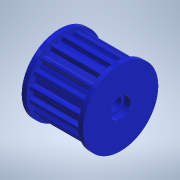
# Autodesk Inventor part: HTPT18S8M300-A-H12_b
Saved by Autodesk Inventor 2021 (Build 250183000, 183)
## iProperties
Category: PARTsolutions
Company: MISUMI
Part Number: HTPT18S8M300-A-H12_b
Material: ABS プラスチック
Catalog Web Link: www.cadenas.de
Description: HTPA__S8M150, HTPA__S8M250, HTPA__S8M300, HTPA__S8M400, HTPB__S8M150, HTPB__S8M250, HTPB__S8M300, HTPB__S8M400, HTPK__S8M150, HTPK__S8M250, HTPK__S8M300, HTPK__S8M400, HTPN__S8M150, HTPN__S8M250, HTPN__S8M300, HTPN__S8M400, HTPT__S8M150, HTPT__S8M250, HTPT__S8M300, HTPT__S8M400, HTPM__S8M150, HTPM__S8M250, HTPM__S8M300, HTPM__S8M400,_body-HTPP__S8M150, HTPP__S8M250, HTPP__S8M300, HTPP__S8M400 - High Torque Timing Pulleys S8M Type
Vendor: MISUMI
Document SubType Name: Modeling
Designer: partserver
Manufacturer: MISUMI
Mass: 50.873 g
Surface Area: 141.05 cm^2
Volume: 47.9934 cm^3
Density: 1.06 g/cm^3
Appearance: 青 - 壁塗料 - 光沢
PSOL_IDENT_0: {$CADENAS_DATA\23d-libs\misumi\metric\51_timing_pulleys\htpa_s8m.prj},749 {VTYP=3D},{NB=HTPT18S8M300
PSOL_IDENT_1: -A-H12_b},{LINA=HTPT18S8M300-A-H12},{NN=HTPA__S8M150, HTPA__S8M250, HTPA__S8M300, HTPA__S8M400, HTPB
PSOL_IDENT_2: __S8M150, HTPB__S8M250, HTPB__S8M300, HTPB__S8M400, HTPK__S8M150, HTPK__S8M250, HTPK__S8M300, HTPK__
PSOL_IDENT_3: S8M400, HTPN__S8M150, HTPN__S8M250, HTPN__S8M300, HTPN__S8M400, HTPT__S8M150, HTPT__S8M250, HTPT__S8
PSOL_IDENT_4: M300, HTPT__S8M400, HTPM__S8M150, HTPM__S8M250, HTPM__S8M300, HTPM__S8M400,_body},{DATE=17.01.2019 0
PSOL_IDENT_5: 4:07:40},{GEOMDATE=11.01.2019 07:18:36},{VERSION=},{LINEID=50},{WBVAR=MATP,ST,TNW,PS,SBS,DD,Z,J,Q,R,
PSOL_IDENT_6: S,T,ALT1,ALT2,M,QSC,QFC,QTC,ALT3,K,KSC,KFC,KTC,ALT4,ZM,ZSC,ZFC,ZTC,ALT5,ALT6,ALT7,FC,ALT8,SRG,ALT9,B
PSOL_IDENT_7: TC,TL,ALT10,TPC,ALT11,BC,ALT12,SLH},{WBNUMERIC=DD,Z,J,Q,R,S,T,QSC,QFC,QTC,K,KSC,KFC,KTC,ZSC,ZFC,ZTC,
PSOL_IDENT_8: FC,SRG,BTC,TL,BC,SLH}  {NB=HTPT18S8M300-A-H12_b},{LINA=HTPT18S8M300-A-H12},{KT=DUMMY},{PN=HTPT18S8M3
PSOL_IDENT_9: 00-A-H12},{TYPE=HTPT},{MATP=S45C},{MATPALG= 'A7075','A7075','S45C','1045 Carbon Steel Equivalent' },
PSOL_IDENT_10: {ST=-},{STALG= '-','-','BO','Black Oxide','ENP','Electroless Nickel Plating' },{NT=18},{TNW=S8M300},
PSOL_IDENT_11: {TNWALG= 'S8M150','S8M250','S8M300','S8M400' },{BW=30},{PS=A},{PSALG= 'A','B' },{SBS=H},{SBSALG= 'H'
PSOL_IDENT_12: ,'Round Hole','P','Round Hole + Tap','N','New JIS Keywayed Bore + Tap (Standard)','C','Old JIS Keywa
PSOL_IDENT_13: yed Bore + Tap','V','Stepped Hole','Y','Both Ends Stepped Hole','WB','Double Stepped Hole' },{DD=12.
PSOL_IDENT_14: 0},{DDALG=12.0,12.7,[13:32/1]},{DDHA=12.0,12.7,[13:32/1]},{DDPA=12.0,12.7,[13:26/1]},{DDNA=[12:26/1]
PSOL_IDENT_15: },{DDCA=[12,15,16,18,19,20]},{DDVA=12.0,12.7,[13:30/1]},{DDY=[12:30/1]},{DDWB=[12:28/1]},{DDHB=},{DD
PSOL_IDENT_16: PB=},{DDNB=},{DDCB=},{DDVFB=},{Z=0},{ZALG=[0]},{ZMIN=14.000},{ZAMAX=32.000},{ZBMAX=0.000},{DDZ=12.00
PSOL_IDENT_17: 0},{J=0.0},{JALG=[0]},{JMIN=3.000},{JMAX=35.000},{JPN=},{Q=0},{QALG=[0]},{QRMIN=14.000},{QRMAX=32.00
PSOL_IDENT_18: 0},{WBQMIN=16.000},{R=0},{RALG=[0]},{WBRMAX=-2.000},{S=0.0},{SALG=[0]},{SMAX=23.000},{T=0.0},{TALG=[
PSOL_IDENT_19: 0]},{TMAX=23.000},{SBSPN=-H12},{A=33},{W=38},{L=0},{PD=45.84},{OD=44.46},{D=0},{DALG=32.000},{DE=36.
PSOL_IDENT_20: 000},{F=52},{E=36},{TT=1.6},{BBK=0.000},{TTK=0.000},{ALT1=},{ALT1ALG= '','Not applicable' },{ANG=120
PSOL_IDENT_21: .000},{ALT1PN=},{ALT2=},{ALT2ALG= '','w/o Side Tapped Hole','QSC','with QSC (6 Places Side Tapped Ho
PSOL_IDENT_22: le)','QFC','with QFC (4 Places Side Tapped Hole)','QTC','with QTC (3 Places Side Tapped Hole)' },{M=
PSOL_IDENT_23: N/A},{MALG= 'N/A' },{MFTALG= 'N/A' },{MSALG= 'N/A' },{M3D=0.000},{KDML=0.000},{ML=0.000},{MUL=0.000}
PSOL_IDENT_24: ,{PITCH=0.000},{QSC=0.0},{QSCALG=0},{QFC=0.0},{QFCALG=0},{QTC=0.0},{QTCALG=0},{QPCDMIN=0.000},{QPCDM
PSOL_IDENT_25: INALG=0.000},{QPCDMAX=32.000},{ALT2PN=},{TAP=0.000},{ALT3=},{ALT3ALG= '','w/o Side Through Hole','KS
PSOL_IDENT_26: C','with KSC (6 Places Side Through Hole)','KFC','with KFC (4 Places Side Through Hole)','KTC','with
PSOL_IDENT_27: KTC (3 Places Side Through Hole)' },{K=0.0},{KALG=0},{KMIN=4.000},{KFTMAX=8.000},{KSMAX=8.000},{KSC=
PSOL_IDENT_28: 0.0},{KSCALG=0},{KFC=0.0},{KFCALG=0},{KTC=0.0},{KTCALG=0},{KSCMIN=16.000},{KPCDMIN=16.000},{KPCDMAX=
PSOL_IDENT_29: 32.000},{ALT3PN=},{ALT4=},{ALT4ALG= '','w/o Side Counterbored','ZSC','with ZSC (6 Places Side Counte
PSOL_IDENT_30: rbored)','ZFC','with ZFC (4 Places Side Counterbored)','ZTC','with ZTC (3 Places Side Counterbored)'
PSOL_IDENT_31: },{ALT4MIN=22.500},{ALT4MAX=25.500},{ZM=N/A},{ZMALG= 'N/A' },{ZMFTALG= 'N/A' },{ZMSALG= 'N/A' },{ZM
PSOL_IDENT_32: DD1=0.0},{ZMDD2=0.0},{ZMHH=0.0},{ZSC=0.0},{ZSCALG=[0]},{ZFC=0.0},{ZFCALG=[0]},{ZTC=0.0},{ZTCALG=[0]}
PSOL_IDENT_33: ,{ZPCDMIN=0.000},{ZPCDMINALG=0.000},{ZPCDMAX=32.000},{ALT4PN=},{ALT5=},{ALT5ALG= '','w/o Flange not
PSOL_IDENT_34: Attached','NFC','with NFC (Flange not Attached)' },{ALT5PN=},{ALT6=},{ALT6ALG= '','w/o Flange Attach
PSOL_IDENT_35: ed on One Side Only','RFC','with RFC (Flange Attached on The Boss Side Only)','LFC','with LFC (Flang
PSOL_IDENT_36: e Attached on The Opposite Side Only)' },{ALT6PN=},{ALT7=},{ALT7ALG= '','w/o FC (Flange Cut)','FC','
PSOL_IDENT_37: with FC (Flange Cut)' },{FC=0.0},{FCALG=0},{FCMIN=45.5},{FCMAX=50.0},{ALT7PN=},{ALT8=},{ALT8ALG= '','
PSOL_IDENT_38: Not applicable' },{ALT8ALGALG=32.000},{ALT8DD2=0.000},{ALT8MM=0.000},{ALT8NN=0.000},{QC=0.000},{KC=0
PSOL_IDENT_39: .000},{ZC=0.000},{SRG=0.0},{SRGALG=[0]},{SRGMAX=0.000},{DD2=0.0},{MM=0.00},{NN=0.00},{ALT8PN=},{ALT9=
PSOL_IDENT_40: },{ALT9ALG= '','w/o BTC (Taper for Bearing Holder)','BTC','with BTC (Taper for Bearing Holder)' },{B
PSOL_IDENT_41: TC9=14.000},{TL9=1.000},{BTC=0},{BTCALG=[0]},{TL=0.0},{TLALG=0},{TLMIN=1.000},{TLMAX=-38.500},{BTCL=
PSOL_IDENT_42: 0},{BTCD=0},{ALT9PN=},{WLBCTL=38.000},{ALT10=},{ALT10ALG= '','Not applicable' },{TPC=N/A},{TPCALG= '
PSOL_IDENT_43: N/A' },{TPCM=4.000},{ALT10PN=},{ALT11=},{ALT11ALG= '','Not applicable' },{BC=0.0},{BCALG=0},{BCMIN=3
PSOL_IDENT_44: .000},{BCMAX=-38.500},{M1WBC=19.000},{ALT11PN=},{KTT=16.230},{ALT12=},{ALT12ALG= '','Not applicable'
PSOL_IDENT_45: },{SLH=0},{SLHALG=[0]},{ALT12PN=},{AC=-},{M1=4.000},{M1L=3.000}
NB: HTPT18S8M300-A-H12_b
NN: 0
NT: 18
NBSYN: $PN._b
LINA: HTPT18S8M300-A-H12
CATALOG: Misumi
PN: HTPT18S8M300-A-H12
MATP: 1045 Carbon Steel Equivalent
ST: -
TNW: S8M300
BW: 30
PS: A
SBS: Round Hole
DD: 12
Z: 0
J: 0
Q: 0
R: 0
S: 0
T: 0
A: 33
W: 38
L: 0
PD: 45.84
OD: 44.46
D: 0
F: 52
E: 36
TT: 1.6
ALT1: Not applicable
ALT2: w/o Side Tapped Hole
M: N/A
QSC: 0
QFC: 0
QTC: 0
ALT3: w/o Side Through Hole
K: 0
KSC: 0
KFC: 0
KTC: 0
ALT4: w/o Side Counterbored
ZM: N/A
ZMDD1: 0
ZMDD2: 0
ZMHH: 0
ZSC: 0
ZFC: 0
ZTC: 0
ALT5: w/o Flange not Attached
ALT6: w/o Flange Attached on One Side Only
ALT7: w/o FC (Flange Cut)
FC: 0
ALT8: Not applicable
SRG: 0
DD2: 0
MM: 0
ALT9: w/o BTC (Taper for Bearing Holder)
BTC: 0
TL: 0
BTCL: 0
BTCD: 0
ALT10: Not applicable
TPC: N/A
ALT11: Not applicable
BC: 0
ALT12: Not applicable
SLH: 0
AC: -
SUPPLIER: MISUMI
ARTICLENO: HTPT18S8M300-A-H12_b
BOMINFO: HTPT18S8M300-A-H12
CREATOR: CADENAS GmbH
Title: HTPT18S8M300-A-H12
Author: Cadenas PARTsolutions
Comments: HTPP__S8M150, HTPP__S8M250, HTPP__S8M300, HTPP__S8M400 - High Torque Timing Pulleys S8M Type
Autodesk Inventor part; units mm, degrees
note: some values were not read from the file. Chosen so that the rebuilt part matches the saved one: pattern direction of "Circular Pattern1".
ref_plane "YZ Plane" through (0, 0, 0) normal (1, 0, 0) x (0, 1, 0)
ref_plane "XZ Plane" through (0, 0, 0) normal (0, 1, 0) x (-1, 0, 0)
ref_plane "XY Plane" through (0, 0, 0) normal (0, 0, 1) x (1, 0, 0)
sketch "_____2" plane through (0, 0, 0) normal (0, 0, 1) x (1, 0, 0)
  line L0 (38, 0) -> (0, 0)
  line L1 (0, 0) -> (0, 18)
  line L2 (0, 18) -> (0.9, 18)
  line L3 (0.9, 18) -> (0.9, 22.0194)
  line L4 (0.9, 22.0194) -> (-0.0556, 25.5859)
  line L5 (-0.0556, 25.5859) -> (1.4898, 26)
  line L6 (1.4898, 26) -> (2.5, 22.23)
  line L7 (2.5, 22.23) -> (35.5, 22.23)
  line L8 (35.5, 22.23) -> (36.5102, 26)
  line L9 (36.5102, 26) -> (38.0556, 25.5859)
  line L10 (38.0556, 25.5859) -> (37.1, 22.0194)
  line L11 (37.1, 22.0194) -> (37.1, 18)
  line L12 (37.1, 18) -> (38, 18)
  line L13 (38, 18) -> (38, 0)
  line L14 (38, 0) -> (0, 0)
  constraints: 30 end point
revolve "Revolution1" add sketch "_____2" angle 360 about axis through (38, 0, 0) along (1, 0, 0)
sketch "Sketch2" plane through (38, 0, 0) normal (1, 0, 0) x (0, 0, -1)
  point P0 (0, 0)
hole "Hole1" at (38, 0, 0) direction (-1, 0, 0) diameter 12 depth 38
sketch "_____6" plane through (2.5, 0, 0) normal (1, 0, 0) x (0, 0, -1)
  arc A0 (-2.5255, 21.4234) -> (-3.3644, 21.9739) centre (-3.2509, 21.2326) ccw
  arc A1 (-2.5255, 21.4234) -> (-1.5801, 19.5137) centre (2.6, 22.7721) ccw
  arc A2 (-1.5801, 19.5137) -> (-1.239, 19.3604) centre (-1.2646, 19.7596) ccw
  arc A3 (1.239, 19.3604) -> (-1.239, 19.3604) centre (0, 0) ccw
  arc A4 (1.239, 19.3604) -> (1.5801, 19.5137) centre (1.2646, 19.7596) ccw
  arc A5 (1.5801, 19.5137) -> (2.5255, 21.4234) centre (-2.6, 22.7721) ccw
  arc A6 (3.3644, 21.9739) -> (2.5255, 21.4234) centre (3.2509, 21.2326) ccw
  line L0 (3.3644, 21.9739) -> (3.3644, 22.6717)
  arc A7 (3.3644, 22.6717) -> (-3.3644, 22.6717) centre (0, 0) ccw
  line L1 (-3.3644, 22.6717) -> (-3.3644, 21.9739)
  constraints: 16 point on circle, 8 centre point, 4 end point
extrude "Extrusion1" cut sketch "_____6" along normal blind 33
pattern_circular "Circular Pattern1" count 18 over 360 about axis through (2.5, 0, 0) along (1, 0, 0) of "Extrusion1"
sketch "スケッチ4" plane through (2.5, 0, 0) normal (1, 0, 0) x (0, 0, -1)
  circle A0 centre (0, 0) radius 26
  circle A1 centre (0, 0) radius 26 projected
  circle A2 centre (0, 0) radius 6 projected
  circle A3 centre (0, 0) radius 6
  constraints: 2 centre point, 2 coincident, 2 concentric
extrude "押し出し2" add sketch "スケッチ4" against normal blind 3
sketch "スケッチ5" plane through (35.5, 0, 0) normal (-1, 0, 0) x (0, -0.3420201, 0.9396926)
  circle A0 centre (0, 0) radius 26
  circle A1 centre (0, 0) radius 26 projected
  circle A2 centre (0, 0) radius 6
  circle A3 centre (0, 0) radius 6 projected
  constraints: 2 centre point, 2 coincident, 2 concentric
extrude "押し出し3" add sketch "スケッチ5" against normal blind 3
sketch "スケッチ6" plane through (38.5, 0, 0) normal (1, 0, 0) x (0, 0, -1)
  circle A0 centre (0, 0) radius 6.25
  dimension "d17" = 12.5
  constraints: 1 centre point, 1 coincident
  measures "d17" diameter of A0
extrude "押し出し4" cut sketch "スケッチ6" against normal blind 4
sketch "スケッチ7" plane through (-0.5, 0, 0) normal (-1, 0, 0) x (0, 0, 1)
  circle A0 centre (0, 0) radius 6.25
  circle A1 centre (0, 0) radius 6.25 projected
  constraints: 1 centre point, 1 coincident, 1 concentric
extrude "押し出し5" cut sketch "スケッチ7" against normal blind 4
sketch "スケッチ8" plane through (34.5, 0, 0) normal (1, 0, 0) x (0, 0, -1)
  circle A0 centre (0, 0) radius 6 projected
  circle A1 centre (0, 0) radius 4.4
  dimension "d23" = 8.8
  constraints: 1 centre point, 1 coincident
  measures "d23" diameter of A1
extrude "押し出し6" add sketch "スケッチ8" against normal up to surface (31 mm away)
sketch "スケッチ9" plane through (38.5, 0, 0) normal (1, 0, 0) x (0, 0, -1)
  circle A0 centre (0, 0) radius 24
  circle A1 centre (0, 0) radius 26 projected
  dimension "d26" = 48
  constraints: 1 centre point, 1 coincident
  measures "d26" diameter of A0
extrude "押し出し7" cut sketch "スケッチ9" against normal through all
body "Solid1"
